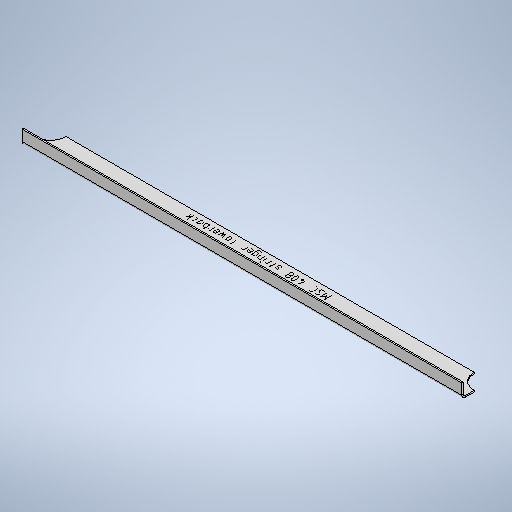
# Autodesk Inventor part: MSC 408 stringer lowerback
Saved by Autodesk Inventor 2025 (Build 290162010, 162A)
## iProperties
Created: 2024-04-28
Part Number: MSC 408 stringer lowerback
Material: Stainless Steel
Document SubType Name: Sheet Metal
Designer: admin
Stock Number: МОО 408 стрингер поясница
Density: 8 g/cm^3
Flat Pattern Width: 62.5 cm
Flat Pattern Length: 5.6202 cm
Flat Pattern Area: 351.262 cm^2
Sheet Metal Rule: AISI304 2mm Die16
Sheet Metal Width: 625,000 mm
Sheet Metal Length: 56,202 mm
Sheet Metal Area: 35126,244 mm^2
Appearance: Default
Author: admin
Autodesk Inventor part; units mm, degrees
ref_plane "YZ Plane" through (0, 0, 0) normal (1, 0, 0) x (0, 1, 0)
ref_plane "XZ Plane" through (0, 0, 0) normal (0, 1, 0) x (-1, 0, 0)
ref_plane "XY Plane" through (0, 0, 0) normal (0, 0, 1) x (1, 0, 0)
sketch "Sketch1" plane through (0, 0, 0) normal (0, 0, 1) x (1, 0, 0)
  line L0 (-312.5, 40) -> (312.5, 40)
  line L1 (312.5, 40) -> (312.5, 0)
  line L2 (312.5, 0) -> (-312.5, 0)
  line L3 (-312.5, 0) -> (-312.5, 40)
  point P0 (0, 0)
  point P1 (0, 0)
  dimension "d1" = 40
  dimension "d45" = 625
  measures "d1" distance of L0.end L1.end
  measures "d45" distance of L1.end L2.end
extrude "Plate1" add sketch "Sketch1" along normal blind 2
sketch "Sketch2" plane through (312.5, 2, 0) normal (0, -1, 0) x (1, 0, 0)
  line L0 (-625, 0) -> (0, 0)
  line L1 (0, 0) -> (0, 20)
  line L2 (0, 20) -> (-625, 20)
  line L3 (-625, 20) -> (-625, 0)
  constraints: 6 end point, 1 horizontal, 1 perpendicular, 1 vertical
edge flange "Flange1" height 20 angle 90 thickness 2 bend radius 2.75 thickness toward (0, -1, 0) relief round relief width 2 relief depth 1 edges at (0, 0, 2) wall of the first edge with corners at (-312.5, 2, 0) (312.5, 2, 0) (312.5, 2, 20) (-312.5, 2, 20)
bend "Bend1"
corner "Corner1"
sketch "Sketch6" plane through (0, 0, 0) normal (0, 0, -1) x (-1, 0, 0)
  line L0 (-312.5, 40) -> (-312.5, 4.75) projected
  circle A0 centre (-312.5, 40) radius 22.5
  line L1 (-312.5, 40) -> (312.5, 40) projected
  line L2 (-499, 30) -> (-499, 67.6691) projected
  point P0 (0, 0)
  point P1 (-290, 40)
  point P2 (-312.5, 17.5)
  point P3 (312.5, 40)
  dimension "d24" = 45
  constraints: 1 centre point, 1 other
  measures "d24" diameter of A0
extrude "Extrusion2" cut sketch "Sketch6" along normal mid plane 30 contours L1 A0 L0 picked at (-297.688, 38.3311)
sketch "Sketch9" plane through (0, 0, 2) normal (0, 0, 1) x (1, 0, 0)
  line L0 (95.482, 35) -> (95.482, 23) construction
  line L1 (95.482, 23) -> (-104.518, 23) construction
  line L2 (-104.518, 23) -> (-104.518, 35) construction
  line L3 (-104.518, 35) -> (95.482, 35) construction
  line L4 (-312.5, 40) -> (312.5, 40) projected
  point P0 (0, 0)
  dimension "d40" = 200
  dimension "d41" = 12
  dimension "d43" = 5
  constraints: 2 other
  measures "d40" distance of L0.end L1.end
  measures "d41" distance of L1.end L2.end
  measures "d43" distance between parallel lines of L4 L3
mark "Mark2"
mirror "Mirror3" about plane through (0, 0, 0) normal (1, 0, 0) of "Extrusion2"
equation "\"d43\" = d42"
equation "\"d2\" = Thickness"
equation "\"d3\" = BendReliefWidth"
equation "\"d4\" = BendReliefDepth"
equation "\"d5\" = MinimumRemnant"
equation "\"d6\" = TransitionRadius"
equation "\"d9\" = BendRadius"
equation "\"d10\" = CornerReliefSize"
equation "\"d11\" = GapSize"
equation "\"d12\" = JacobiRadiusSize"
equation "\"BendReliefWidth\" = Thickness"
equation "\"BendReliefDepth\" = 0.5 * Thickness"
equation "\"CornerReliefSize\" = 4 * Thickness"
equation "\"MinimumRemnant\" = 2 * Thickness"
equation "\"TransitionRadius\" = BendRadius"
equation "\"JacobiRadiusSize\" = BendRadius"
equation "\"GapSize\" = Thickness"
equation "\"qqqqqq\" = 67.35706"
equation "\"d42\" = 5"
equation "\"Thickness\" = 2"
equation "\"BendRadius\" = 2.75"
body "Solid1"
